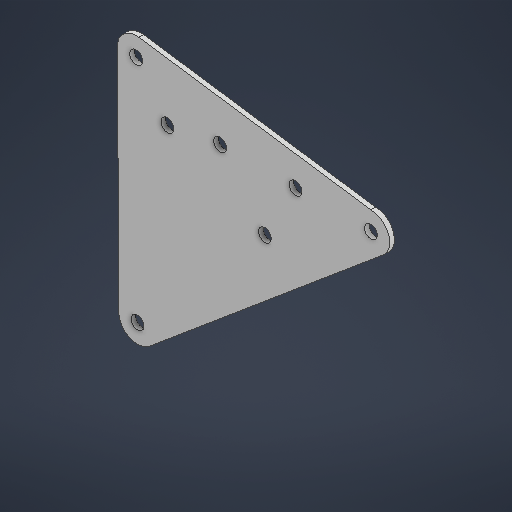
# Autodesk Inventor part: Lbsupportpoly
Saved by Autodesk Inventor 2025.2 (Build 292293000, 293)
## iProperties
Created: 2025-03-29
Part Number: Lbsupportpoly
Material: Generic
Document SubType Name: Modeling
Designer: roejo
Density: 1 g/cm^3
Appearance: Default
Author: roejo
Autodesk Inventor part; units mm, degrees
ref_plane "YZ Plane" through (0, 0, 0) normal (1, 0, 0) x (0, 1, 0)
ref_plane "XZ Plane" through (0, 0, 0) normal (0, 1, 0) x (-1, 0, 0)
ref_plane "XY Plane" through (0, 0, 0) normal (0, 0, 1) x (1, 0, 0)
sketch "Sketch1" plane through (0, 0, 0) normal (0, 0, 1) x (1, 0, 0)
  circle A0 centre (-19.9771, 22.6292) radius 2.1844
  circle A1 centre (-37.7835, 19.4142) radius 2.1844
  circle A2 centre (-48.3036, 33.9712) radius 2.1844
  circle A3 centre (-4.9059, 3.7677) radius 2.1844
  circle A4 centre (5.4229, 22.6292) radius 2.1844
  circle A5 centre (-47.8758, -43.2787) radius 2.1844
  circle A6 centre (-4.9059, 3.7677) radius 6.35
  circle A7 centre (5.4229, 22.6292) radius 6.35
  circle A8 centre (-19.9771, 22.6292) radius 6.35
  circle A9 centre (-48.3036, 33.9712) radius 6.35
  circle A10 centre (-47.8758, -43.2787) radius 6.35
  circle A11 centre (30.8229, 22.6292) radius 2.1844
  circle A12 centre (30.8229, 22.6292) radius 6.35
  circle A13 centre (-37.7835, 19.4142) radius 6.35
  line L0 (30.8229, 28.9792) -> (-47.3975, 40.2562)
  line L1 (-54.2258, -43.2787) -> (-54.5729, 34.9804)
  line L2 (34.1649, 17.2298) -> (-43.7957, -48.1444)
  point P0 (0, 0)
  dimension "d0" = 12.7
  dimension "d1" = 12.7
  dimension "d2" = 12.7
  dimension "d3" = 12.7
  dimension "d4" = 12.7
  dimension "d5" = 12.7
  dimension "d6" = 12.7
  constraints: 14 centre point, 7 coincident, 6 end point, 6 point on circle, 2 tangent
  measures "d0" diameter of A6
  measures "d1" diameter of A7
  measures "d2" diameter of A8
  measures "d3" diameter of A9
  measures "d4" diameter of A10
  measures "d5" diameter of A12
  measures "d6" diameter of A13
extrude "Extrusion1" add sketch "Sketch1" along normal blind 1.5875 contours A6 | A7 | A8 | A9 L1 | A9 L0 A12 L2 A10 L1 | A12 | A10 | A13 picked at (-53.2082, 33.9527)
body "Solid1"
